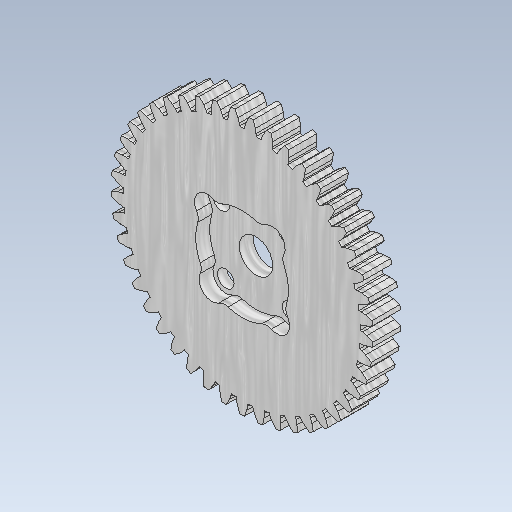
# Autodesk Inventor part: m1歯数45同軸ギア5td6
Saved by Autodesk Inventor 2020.2 (Build 242310000, 310)
## iProperties
Created: 2020-02-29
Part Number: m1歯数45同軸ギア5td6
Material: アルミニウム 7075
Document SubType Name: Modeling
Designer: aoyam
Density: 2.81 g/cm^3
Appearance: サテン - ブラシ仕上げ 重厚
Author: aoyam
Autodesk Inventor part; units mm, degrees
ref_plane "YZ Plane" through (0, 0, 0) normal (1, 0, 0) x (0, 1, 0)
ref_plane "XZ Plane" through (0, 0, 0) normal (0, 1, 0) x (-1, 0, 0)
ref_plane "XY Plane" through (0, 0, 0) normal (0, 0, 1) x (1, 0, 0)
sketch "スケッチ1" plane through (0, 0, 0) normal (0, 0, 1) x (1, 0, 0)
  arc A0 (1.8358, 22.8336) -> (1.7596, 22.4335) centre (5.1577, 21.9932) ccw
  arc A1 (2.0665, 23.5562) -> (1.8358, 22.8336) centre (7.6641, 21.3711) ccw
  arc A2 (2.5802, 24.6469) -> (2.0665, 23.5562) centre (10.2505, 20.3678) ccw
  arc A3 (0.898, 22.4335) -> (0.8218, 22.8336) centre (-2.5001, 21.9932) ccw
  arc A4 (0.8218, 22.8336) -> (0.5911, 23.5562) centre (-5.0065, 21.3711) ccw
  arc A5 (0.5911, 23.5562) -> (0.0774, 24.6469) centre (-7.5929, 20.3678) ccw
  arc A6 (1.7596, 22.4335) -> (0.898, 22.4335) centre (1.3288, 1.2587) ccw
  arc A7 (0.0774, 24.6469) -> (-0.687, 24.5934) centre (1.3288, 1.2587) ccw
  arc A8 (-1.1916, 22.2873) -> (-2.0447, 22.1674) centre (1.3288, 1.2587) ccw
  arc A9 (-2.0447, 22.1674) -> (-2.176, 22.5531) centre (-5.3485, 21.2585) ccw
  arc A10 (-1.1718, 22.6942) -> (-1.1916, 22.2873) centre (2.2347, 22.3243) ccw
  arc A11 (-2.176, 22.5531) -> (-2.505, 23.2366) centre (-7.744, 20.2937) ccw
  arc A12 (-1.0439, 23.4419) -> (-1.1718, 22.6942) centre (4.8033, 22.0571) ccw
  arc A13 (-0.687, 24.5934) -> (-1.0439, 23.4419) centre (7.5042, 21.4234) ccw
  arc A14 (-2.505, 23.2366) -> (-3.1655, 24.2451) centre (-10.1655, 18.9401) ccw
  arc A15 (-3.1655, 24.2451) -> (-3.9149, 24.0858) centre (1.3288, 1.2587) ccw
  arc A16 (-4.0937, 21.7319) -> (-4.9218, 21.4944) centre (1.3288, 1.2587) ccw
  arc A17 (-4.9218, 21.4944) -> (-5.1055, 21.8581) centre (-8.0669, 20.1346) ccw
  arc A18 (-4.1307, 22.1376) -> (-4.0937, 21.7319) centre (-0.7059, 22.2453) ccw
  arc A19 (-5.1055, 21.8581) -> (-5.5264, 22.4891) centre (-10.3048, 18.8457) ccw
  arc A20 (-4.1081, 22.8958) -> (-4.1307, 22.1376) centre (1.8749, 22.3382) ccw
  arc A21 (-3.9149, 24.0858) -> (-4.1081, 22.8958) centre (4.6377, 22.0867) ccw
  arc A22 (-5.5264, 22.4891) -> (-6.3208, 23.3959) centre (-12.5145, 17.1684) ccw
  arc A23 (-6.3208, 23.3959) -> (-7.0408, 23.1339) centre (1.3288, 1.2587) ccw
  arc A24 (-6.8902, 20.778) -> (-7.6773, 20.4276) centre (1.3288, 1.2587) ccw
  arc A25 (-7.6773, 20.4276) -> (-7.9097, 20.7621) centre (-10.6025, 18.6432) ccw
  arc A26 (-6.9833, 21.1746) -> (-6.8902, 20.778) centre (-3.6069, 21.7579) ccw
  arc A27 (-7.9097, 20.7621) -> (-8.4144, 21.3284) centre (-12.6393, 17.0555) ccw
  arc A28 (-7.0665, 21.9286) -> (-6.9833, 21.1746) centre (-1.0641, 22.2091) ccw
  arc A29 (-7.0408, 23.1339) -> (-7.0665, 21.9286) centre (1.7068, 22.3445) ccw
  arc A30 (-8.4144, 21.3284) -> (-9.3273, 22.1159) centre (-14.5939, 15.0869) ccw
  arc A31 (-9.3273, 22.1159) -> (-10.0038, 21.7562) centre (1.3288, 1.2587) ccw
  arc A32 (-9.5268, 19.4442) -> (-10.2574, 18.9876) centre (1.3288, 1.2587) ccw
  arc A33 (-10.2574, 18.9876) -> (-10.5342, 19.2866) centre (-12.9059, 16.8135) ccw
  arc A34 (-9.6742, 19.824) -> (-9.5268, 19.4442) centre (-6.4118, 20.8715) ccw
  arc A35 (-10.5342, 19.2866) -> (-11.1127, 19.7771) centre (-14.7018, 14.9578) ccw
  arc A36 (-9.8615, 20.559) -> (-9.6742, 19.824) centre (-3.9565, 21.6722) ccw
  arc A37 (-10.0038, 21.7562) -> (-9.8615, 20.559) centre (-1.2315, 22.1919) ccw
  arc A38 (-11.1127, 19.7771) -> (-12.1263, 20.4298) centre (-16.3635, 12.7363) ccw
  arc A39 (-12.1263, 20.4298) -> (-12.7462, 19.9795) centre (1.3288, 1.2587) ccw
  arc A40 (-11.9521, 17.7564) -> (-12.6121, 17.2026) centre (1.3288, 1.2587) ccw
  arc A41 (-12.6121, 17.2026) -> (-12.9277, 17.4601) centre (-14.9322, 14.6811) ccw
  arc A42 (-12.1509, 18.112) -> (-11.9521, 17.7564) centre (-9.066, 19.6034) ccw
  arc A43 (-12.9277, 17.4601) -> (-13.5689, 17.8654) centre (-16.4524, 12.5934) ccw
  arc A44 (-12.4387, 18.8138) -> (-12.1509, 18.112) centre (-6.7461, 20.7379) ccw
  arc A45 (-12.7462, 19.9795) -> (-12.4387, 18.8138) centre (-4.1199, 21.6318) ccw
  arc A46 (-13.5689, 17.8654) -> (-14.6635, 18.3707) centre (-17.7887, 10.1623) ccw
  arc A47 (-14.6635, 18.3707) -> (-15.2147, 17.8384) centre (1.3288, 1.2587) ccw
  arc A48 (-14.1189, 15.7475) -> (-14.6954, 15.1072) centre (1.3288, 1.2587) ccw
  arc A49 (-14.6954, 15.1072) -> (-15.0438, 15.3183) centre (-16.642, 12.2874) ccw
  arc A50 (-14.3653, 16.0719) -> (-14.1189, 15.7475) centre (-11.5179, 17.9782) ccw
  arc A51 (-15.0438, 15.3183) -> (-15.7352, 15.6304) centre (-17.8568, 10.0085) ccw
  arc A52 (-14.7479, 16.7269) -> (-14.3653, 16.0719) centre (-9.3785, 19.4246) ccw
  arc A53 (-15.2147, 17.8384) -> (-14.7479, 16.7269) centre (-6.9023, 20.6752) ccw
  arc A54 (-15.7352, 15.6304) -> (-16.8894, 15.9784) centre (-18.8418, 7.415) ccw
  arc A55 (-16.8894, 15.9784) -> (-17.3611, 15.3747) centre (1.3288, 1.2587) ccw
  arc A56 (-15.985, 13.4566) -> (-16.4668, 12.7423) centre (1.3288, 1.2587) ccw
  arc A57 (-16.4668, 12.7423) -> (-16.8412, 12.9029) centre (-18.002, 9.679) ccw
  arc A58 (-16.2741, 13.7436) -> (-15.985, 13.4566) centre (-13.7198, 16.0275) ccw
  arc A59 (-16.8412, 12.9029) -> (-17.5693, 13.1157) centre (-18.8878, 7.2532) ccw
  arc A60 (-16.7442, 14.3389) -> (-16.2741, 13.7436) centre (-11.8025, 17.7576) ccw
  arc A61 (-17.3611, 15.3747) -> (-16.7442, 14.3389) centre (-9.5244, 19.3407) ccw
  arc A62 (-17.5693, 13.1157) -> (-18.7607, 13.2997) centre (-19.5023, 4.5479) ccw
  arc A63 (-18.7607, 13.2997) -> (-19.1438, 12.6362) centre (1.3288, 1.2587) ccw
  arc A64 (-17.5141, 10.9283) -> (-17.8918, 10.1539) centre (1.3288, 1.2587) ccw
  arc A65 (-17.8918, 10.1539) -> (-18.2849, 10.2608) centre (-18.9857, 6.9067) ccw
  arc A66 (-17.8404, 11.1722) -> (-17.5141, 10.9283) centre (-15.6288, 13.7894) ccw
  arc A67 (-18.2849, 10.2608) -> (-19.0355, 10.3702) centre (-19.5254, 4.3812) ccw
  arc A68 (-18.3887, 11.6963) -> (-17.8404, 11.1722) centre (-13.9709, 15.7695) ccw
  arc A69 (-19.1438, 12.6362) -> (-18.3887, 11.6963) centre (-11.9353, 17.6543) ccw
  arc A70 (-19.0355, 10.3702) -> (-20.241, 10.3866) centre (-19.7574, 1.6168) ccw
  arc A71 (-20.241, 10.3866) -> (-20.528, 9.6762) centre (1.3288, 1.2587) ccw
  arc A72 (-18.6765, 8.2117) -> (-18.9427, 7.3924) centre (1.3288, 1.2587) ccw
  arc A73 (-18.9427, 7.3924) -> (-19.3469, 7.4435) centre (-19.5741, 4.0245) ccw
  arc A74 (-19.0335, 8.4079) -> (-18.6765, 8.2117) centre (-17.2077, 11.3074) ccw
  arc A75 (-19.3469, 7.4435) -> (-20.1054, 7.4474) centre (-19.757, 1.4485) ccw
  arc A76 (-19.6495, 8.8506) -> (-19.0335, 8.4079) centre (-15.8415, 13.499) ccw
  arc A77 (-20.528, 9.6762) -> (-19.6495, 8.8506) centre (-14.0881, 15.6487) ccw
  arc A78 (-20.1054, 7.4474) -> (-21.3014, 7.2958) centre (-19.602, -1.3213) ccw
  arc A79 (-21.3014, 7.2958) -> (-21.4868, 6.5524) centre (1.3288, 1.2587) ccw
  arc A80 (-19.4495, 5.3599) -> (-19.5991, 4.5114) centre (1.3288, 1.2587) ccw
  arc A81 (-19.5991, 4.5114) -> (-20.0064, 4.5058) centre (-19.7556, 1.0885) ccw
  arc A82 (-19.8303, 5.5044) -> (-19.4495, 5.3599) centre (-18.4258, 8.6299) ccw
  arc A83 (-20.0064, 4.5058) -> (-20.7581, 4.4041) centre (-19.5782, -1.4879) ccw
  arc A84 (-20.5019, 5.8571) -> (-19.8303, 5.5044) centre (-17.378, 10.9902) ccw
  arc A85 (-21.4868, 6.5524) -> (-20.5019, 5.8571) centre (-15.9408, 13.3631) ccw
  arc A86 (-20.7581, 4.4041) -> (-21.9214, 4.0876) centre (-19.0392, -4.2092) ccw
  arc A87 (-21.9214, 4.0876) -> (-22.0015, 3.3256) centre (1.3288, 1.2587) ccw
  arc A88 (-19.8181, 2.4282) -> (-19.8481, 1.5672) centre (1.3288, 1.2587) ccw
  arc A89 (-19.8481, 1.5672) -> (-20.2507, 1.5049) centre (-19.5267, -1.8442) ccw
  arc A90 (-20.2153, 2.5183) -> (-19.8181, 2.4282) centre (-19.2595, 5.8088) ccw
  arc A91 (-20.2507, 1.5049) -> (-20.9809, 1.2996) centre (-18.9925, -4.3709) ccw
  arc A92 (-20.9294, 2.7741) -> (-20.2153, 2.5183) centre (-18.5503, 8.292) ccw
  arc A93 (-22.0015, 3.3256) -> (-20.9294, 2.7741) centre (-17.4573, 10.8418) ccw
  arc A94 (-20.9809, 1.2996) -> (-22.0888, 0.8242) centre (-18.08, -6.9907) ccw
  arc A95 (-22.0888, 0.8242) -> (-22.0621, 0.0585) centre (1.3288, 1.2587) ccw
  arc A96 (-19.775, -0.5263) -> (-19.685, -1.3831) centre (1.3288, 1.2587) ccw
  arc A97 (-19.685, -1.3831) -> (-20.075, -1.5008) centre (-18.8919, -4.7166) ccw
  arc A98 (-20.181, -0.4923) -> (-19.775, -0.5263) centre (-19.6924, 2.8992) ccw
  arc A99 (-20.075, -1.5008) -> (-20.7695, -1.8057) centre (-18.0112, -7.1443) ccw
  arc A100 (-20.9237, -0.3384) -> (-20.181, -0.4923) centre (-19.3357, 5.4569) ccw
  arc A101 (-22.0621, 0.0585) -> (-20.9237, -0.3384) centre (-18.6082, 8.134) ccw
  arc A102 (-20.7695, -1.8057) -> (-21.8005, -2.4306) centre (-16.743, -9.6116) ccw
  arc A103 (-21.8005, -2.4306) -> (-21.6674, -3.1852) centre (1.3288, 1.2587) ccw
  arc A104 (-19.3212, -3.446) -> (-19.1128, -4.2819) centre (1.3288, 1.2587) ccw
  arc A105 (-19.1128, -4.2819) -> (-19.4826, -4.4528) centre (-17.8635, -7.4726) ccw
  arc A106 (-19.728, -3.4688) -> (-19.3212, -3.446) centre (-19.7161, -0.0423) ccw
  arc A107 (-19.4826, -4.4528) -> (-20.128, -4.8514) centre (-16.6536, -9.7541) ccw
  arc A108 (-20.4849, -3.4198) -> (-19.728, -3.4688) centre (-19.7189, 2.5401) ccw
  arc A109 (-21.6674, -3.1852) -> (-20.4849, -3.4198) centre (-19.371, 5.2924) ccw
  arc A110 (-20.128, -4.8514) -> (-21.0619, -5.6137) centre (-15.0543, -12.0209) ccw
  arc A111 (-21.0619, -5.6137) -> (-20.8252, -6.3424) centre (1.3288, 1.2587) ccw
  arc A112 (-18.4655, -6.2741) -> (-18.1428, -7.0729) centre (1.3288, 1.2587) ccw
  arc A113 (-18.1428, -7.0729) -> (-18.4852, -7.2936) centre (-16.4616, -10.0587) ccw
  arc A114 (-18.8651, -6.3533) -> (-18.4655, -6.2741) centre (-19.3302, -2.9586) ccw
  arc A115 (-18.4852, -7.2936) -> (-19.0688, -7.7782) centre (-14.9459, -12.1496) ccw
  arc A116 (-19.6215, -6.4101) -> (-18.8651, -6.3533) centre (-19.6924, -0.4016) ccw
  arc A117 (-20.8252, -6.3424) -> (-19.6215, -6.4101) centre (-19.731, 2.3723) ccw
  arc A118 (-19.0688, -7.7782) -> (-19.8876, -8.663) centre (-13.0467, -14.1718) ccw
  arc A119 (-19.8876, -8.663) -> (-19.5517, -9.3517) centre (1.3288, 1.2587) ccw
  arc A120 (-17.2245, -8.9557) -> (-16.7937, -9.7018) centre (1.3288, 1.2587) ccw
  arc A121 (-16.7937, -9.7018) -> (-17.1022, -9.9679) centre (-14.7134, -12.4245) ccw
  arc A122 (-17.6092, -9.0897) -> (-17.2245, -8.9557) centre (-18.5422, -5.7927) ccw
  arc A123 (-17.1022, -9.9679) -> (-17.6126, -10.529) centre (-12.9214, -14.2841) ccw
  arc A124 (-18.3503, -9.2512) -> (-17.6092, -9.0897) centre (-19.2567, -3.311) ccw
  arc A125 (-19.5517, -9.3517) -> (-18.3503, -9.2512) centre (-19.681, -0.5695) ccw
  arc A126 (-17.6126, -10.529) -> (-18.3003, -11.5192) centre (-10.7593, -16.0223) ccw
  arc A127 (-18.3003, -11.5192) -> (-17.8718, -12.1544) centre (1.3288, 1.2587) ccw
  arc A128 (-15.6224, -11.4384) -> (-15.092, -12.1173) centre (1.3288, 1.2587) ccw
  arc A129 (-15.092, -12.1173) -> (-15.3603, -12.4238) centre (-12.6529, -14.524) ccw
  arc A130 (-15.9847, -11.6247) -> (-15.6224, -11.4384) centre (-17.3675, -8.4896) ccw
  arc A131 (-15.3603, -12.4238) -> (-15.7877, -13.0504) centre (-10.6196, -16.1161) ccw
  arc A132 (-16.6961, -11.8878) -> (-15.9847, -11.6247) centre (-18.4204, -6.1315) ccw
  arc A133 (-17.8718, -12.1544) -> (-16.6961, -11.8878) centre (-19.2221, -3.4757) ccw
  arc A134 (-15.7877, -13.0504) -> (-16.3309, -14.1267) centre (-8.2366, -17.5364) ccw
  arc A135 (-16.3309, -14.1267) -> (-15.8182, -14.6961) centre (1.3288, 1.2587) ccw
  arc A136 (-13.6903, -13.674) -> (-13.0706, -14.2724) centre (1.3288, 1.2587) ccw
  arc A137 (-13.0706, -14.2724) -> (-13.2937, -14.6133) centre (-10.3204, -16.3162) ccw
  arc A138 (-14.0232, -13.9088) -> (-13.6903, -13.674) centre (-15.8289, -10.9967) ccw
  arc A139 (-13.2937, -14.6133) -> (-13.6297, -15.2933) centre (-8.0852, -17.6099) ccw
  arc A140 (-14.6911, -14.2684) -> (-14.0232, -13.9088) centre (-17.1997, -8.8081) ccw
  arc A141 (-15.8182, -14.6961) -> (-14.6911, -14.2684) centre (-18.3632, -6.2897) ccw
  arc A142 (-13.6297, -15.2933) -> (-14.0178, -16.4347) centre (-5.5278, -18.6848) ccw
  arc A143 (-14.0178, -16.4347) -> (-13.4309, -16.9272) centre (1.3288, 1.2587) ccw
  arc A144 (-11.4659, -15.6189) -> (-10.7689, -16.1253) centre (1.3288, 1.2587) ccw
  arc A145 (-10.7689, -16.1253) -> (-10.9425, -16.4939) centre (-7.761, -17.7664) ccw
  arc A146 (-11.7628, -15.8978) -> (-11.4659, -15.6189) centre (-13.9563, -13.2654) ccw
  arc A147 (-10.9425, -16.4939) -> (-11.1806, -17.2141) centre (-5.3676, -18.7364) ccw
  arc A148 (-12.3742, -16.3468) -> (-11.7628, -15.8978) centre (-15.6184, -11.2888) ccw
  arc A149 (-13.4309, -16.9272) -> (-12.3742, -16.3468) centre (-17.121, -8.9569) ccw
  arc A150 (-11.1806, -17.2141) -> (-11.406, -18.3984) centre (-2.6855, -19.4449) ccw
  arc A151 (-11.406, -18.3984) -> (-10.7563, -18.8044) centre (1.3288, 1.2587) ccw
  arc A152 (-8.9925, -17.2353) -> (-8.2318, -17.6398) centre (1.3288, 1.2587) ccw
  arc A153 (-8.2318, -17.6398) -> (-8.3524, -18.0289) centre (-5.0248, -18.8464) ccw
  arc A154 (-9.2477, -17.5529) -> (-8.9925, -17.2353) centre (-11.7861, -15.2513) ccw
  arc A155 (-8.3524, -18.0289) -> (-8.4879, -18.7753) centre (-2.5197, -19.4738) ccw
  arc A156 (-9.7906, -18.0826) -> (-9.2477, -17.5529) centre (-13.7072, -13.5253) ccw
  arc A157 (-10.7563, -18.8044) -> (-9.7906, -18.0826) centre (-15.5198, -11.4252) ccw
  arc A158 (-8.4879, -18.7753) -> (-8.5464, -19.9794) centre (0.235, -19.8021) ccw
  arc A159 (-8.5464, -19.9794) -> (-7.8464, -20.291) centre (1.3288, 1.2587) ccw
  arc A160 (-6.3182, -18.4918) -> (-5.5086, -18.7865) centre (1.3288, 1.2587) ccw
  arc A161 (-5.5086, -18.7865) -> (-5.5738, -19.1886) centre (-2.1649, -19.5349) ccw
  arc A162 (-6.5267, -18.8417) -> (-6.3182, -18.4918) centre (-9.3608, -16.9159) ccw
  arc A163 (-5.5738, -19.1886) -> (-5.6042, -19.9465) centre (0.4032, -19.8076) ccw
  arc A164 (-6.9907, -19.4419) -> (-6.5267, -18.8417) centre (-11.5033, -15.474) ccw
  arc A165 (-7.8464, -20.291) -> (-6.9907, -19.4419) centre (-13.5905, -13.6466) ccw
  arc A166 (-5.6042, -19.9465) -> (-5.4945, -21.1471) centre (3.1767, -19.7494) ccw
  arc A167 (-5.4945, -21.1471) -> (-4.758, -21.3583) centre (1.3288, 1.2587) ccw
  arc A168 (-3.495, -19.3638) -> (-2.6523, -19.543) centre (1.3288, 1.2587) ccw
  arc A169 (-2.6523, -19.543) -> (-2.6609, -19.9502) centre (0.763, -19.8188) ccw
  arc A170 (-3.6528, -19.7394) -> (-3.495, -19.3638) centre (-6.7273, -18.2267) ccw
  arc A171 (-2.6609, -19.9502) -> (-2.5855, -20.705) centre (3.344, -19.7314) ccw
  arc A172 (-4.0287, -20.3983) -> (-3.6528, -19.7394) centre (-9.0497, -17.0971) ccw
  arc A173 (-4.758, -21.3583) -> (-4.0287, -20.3983) centre (-11.3709, -15.5779) ccw
  arc A174 (-2.5855, -20.705) -> (-2.3098, -21.8786) centre (6.0825, -19.2878) ccw
  arc A175 (-2.3098, -21.8786) -> (-1.5511, -21.9853) centre (1.3288, 1.2587) ccw
  arc A176 (-0.578, -19.8345) -> (0.2814, -19.8946) centre (1.3288, 1.2587) ccw
  arc A177 (0.2814, -19.8946) -> (0.3296, -20.2991) centre (3.702, -19.6924) ccw
  arc A178 (-0.682, -20.2284) -> (-0.578, -19.8345) centre (-3.9371, -19.1582) ccw
  arc A179 (0.3296, -20.2991) -> (0.5093, -21.036) centre (6.2457, -19.2467) ccw
  arc A180 (-0.9625, -20.9331) -> (-0.682, -20.2284) centre (-6.394, -18.3628) ccw
  arc A181 (-1.5511, -21.9853) -> (-0.9625, -20.9331) centre (-8.9041, -17.1815) ccw
  arc A182 (0.5093, -21.036) -> (0.9457, -22.1599) centre (8.8958, -18.4262) ccw
  arc A183 (0.9457, -22.1599) -> (1.7119, -22.1599) centre (1.3288, 1.2587) ccw
  arc A184 (2.3762, -19.8946) -> (3.2356, -19.8345) centre (1.3288, 1.2587) ccw
  arc A185 (3.2356, -19.8345) -> (3.3396, -20.2284) centre (6.5947, -19.1582) ccw
  arc A186 (2.328, -20.2991) -> (2.3762, -19.8946) centre (-1.0444, -19.6924) ccw
  arc A187 (3.3396, -20.2284) -> (3.6201, -20.9331) centre (9.0516, -18.3628) ccw
  arc A188 (2.1483, -21.036) -> (2.328, -20.2991) centre (-3.5881, -19.2467) ccw
  arc A189 (1.7119, -22.1599) -> (2.1483, -21.036) centre (-6.2382, -18.4262) ccw
  arc A190 (3.6201, -20.9331) -> (4.2087, -21.9853) centre (11.5617, -17.1815) ccw
  arc A191 (4.2087, -21.9853) -> (4.9674, -21.8786) centre (1.3288, 1.2587) ccw
  arc A192 (5.3099, -19.543) -> (6.1526, -19.3638) centre (1.3288, 1.2587) ccw
  arc A193 (6.1526, -19.3638) -> (6.3104, -19.7394) centre (9.3849, -18.2267) ccw
  arc A194 (5.3185, -19.9502) -> (5.3099, -19.543) centre (1.8946, -19.8188) ccw
  arc A195 (6.3104, -19.7394) -> (6.6863, -20.3983) centre (11.7073, -17.0971) ccw
  arc A196 (5.2431, -20.705) -> (5.3185, -19.9502) centre (-0.6865, -19.7314) ccw
  arc A197 (4.9674, -21.8786) -> (5.2431, -20.705) centre (-3.4249, -19.2878) ccw
  arc A198 (6.6863, -20.3983) -> (7.4156, -21.3583) centre (14.0285, -15.5779) ccw
  arc A199 (7.4156, -21.3583) -> (8.1521, -21.1471) centre (1.3288, 1.2587) ccw
  arc A200 (8.1662, -18.7865) -> (8.9758, -18.4918) centre (1.3288, 1.2587) ccw
  arc A201 (8.9758, -18.4918) -> (9.1843, -18.8417) centre (12.0184, -16.9159) ccw
  arc A202 (8.2314, -19.1886) -> (8.1662, -18.7865) centre (4.8225, -19.5349) ccw
  arc A203 (9.1843, -18.8417) -> (9.6482, -19.4419) centre (14.1609, -15.474) ccw
  arc A204 (8.2618, -19.9465) -> (8.2314, -19.1886) centre (2.2544, -19.8076) ccw
  arc A205 (8.1521, -21.1471) -> (8.2618, -19.9465) centre (-0.5191, -19.7494) ccw
  arc A206 (9.6482, -19.4419) -> (10.504, -20.291) centre (16.2481, -13.6466) ccw
  arc A207 (10.504, -20.291) -> (11.2039, -19.9794) centre (1.3288, 1.2587) ccw
  arc A208 (10.8894, -17.6398) -> (11.6501, -17.2353) centre (1.3288, 1.2587) ccw
  arc A209 (11.6501, -17.2353) -> (11.9053, -17.5529) centre (14.4437, -15.2513) ccw
  arc A210 (11.0099, -18.0289) -> (10.8894, -17.6398) centre (7.6824, -18.8464) ccw
  arc A211 (11.9053, -17.5529) -> (12.4482, -18.0826) centre (16.3648, -13.5253) ccw
  arc A212 (11.1455, -18.7753) -> (11.0099, -18.0289) centre (5.1773, -19.4738) ccw
  arc A213 (11.2039, -19.9794) -> (11.1455, -18.7753) centre (2.4226, -19.8021) ccw
  arc A214 (12.4482, -18.0826) -> (13.4138, -18.8044) centre (18.1773, -11.4252) ccw
  arc A215 (13.4138, -18.8044) -> (14.0636, -18.3984) centre (1.3288, 1.2587) ccw
  arc A216 (13.4265, -16.1253) -> (14.1235, -15.6189) centre (1.3288, 1.2587) ccw
  arc A217 (14.1235, -15.6189) -> (14.4204, -15.8978) centre (16.6138, -13.2654) ccw
  arc A218 (13.6, -16.4939) -> (13.4265, -16.1253) centre (10.4186, -17.7664) ccw
  arc A219 (14.4204, -15.8978) -> (15.0318, -16.3468) centre (18.276, -11.2888) ccw
  arc A220 (13.8381, -17.2141) -> (13.6, -16.4939) centre (8.0252, -18.7364) ccw
  arc A221 (14.0636, -18.3984) -> (13.8381, -17.2141) centre (5.343, -19.4449) ccw
  arc A222 (15.0318, -16.3468) -> (16.0885, -16.9272) centre (19.7786, -8.9569) ccw
  arc A223 (16.0885, -16.9272) -> (16.6754, -16.4347) centre (1.3288, 1.2587) ccw
  arc A224 (15.7282, -14.2724) -> (16.3479, -13.674) centre (1.3288, 1.2587) ccw
  arc A225 (16.3479, -13.674) -> (16.6807, -13.9088) centre (18.4864, -10.9967) ccw
  arc A226 (15.9513, -14.6133) -> (15.7282, -14.2724) centre (12.9779, -16.3162) ccw
  arc A227 (16.6807, -13.9088) -> (17.3487, -14.2684) centre (19.8573, -8.8081) ccw
  arc A228 (16.2873, -15.2933) -> (15.9513, -14.6133) centre (10.7428, -17.6099) ccw
  arc A229 (16.6754, -16.4347) -> (16.2873, -15.2933) centre (8.1854, -18.6848) ccw
  arc A230 (17.3487, -14.2684) -> (18.4758, -14.6961) centre (21.0208, -6.2897) ccw
  arc A231 (18.4758, -14.6961) -> (18.9885, -14.1267) centre (1.3288, 1.2587) ccw
  arc A232 (17.7495, -12.1173) -> (18.28, -11.4384) centre (1.3288, 1.2587) ccw
  arc A233 (18.28, -11.4384) -> (18.6423, -11.6247) centre (20.0251, -8.4896) ccw
  arc A234 (18.0179, -12.4238) -> (17.7495, -12.1173) centre (15.3105, -14.524) ccw
  arc A235 (18.6423, -11.6247) -> (19.3537, -11.8878) centre (21.078, -6.1315) ccw
  arc A236 (18.4453, -13.0504) -> (18.0179, -12.4238) centre (13.2772, -16.1161) ccw
  arc A237 (18.9885, -14.1267) -> (18.4453, -13.0504) centre (10.8942, -17.5364) ccw
  arc A238 (19.3537, -11.8878) -> (20.5294, -12.1544) centre (21.8797, -3.4757) ccw
  arc A239 (20.5294, -12.1544) -> (20.9579, -11.5192) centre (1.3288, 1.2587) ccw
  arc A240 (19.4513, -9.7018) -> (19.8821, -8.9557) centre (1.3288, 1.2587) ccw
  arc A241 (19.8821, -8.9557) -> (20.2668, -9.0897) centre (21.1998, -5.7927) ccw
  arc A242 (19.7597, -9.9679) -> (19.4513, -9.7018) centre (17.371, -12.4245) ccw
  arc A243 (20.2668, -9.0897) -> (21.0079, -9.2512) centre (21.9143, -3.311) ccw
  arc A244 (20.2702, -10.529) -> (19.7597, -9.9679) centre (15.579, -14.2841) ccw
  arc A245 (20.9579, -11.5192) -> (20.2702, -10.529) centre (13.4169, -16.0223) ccw
  arc A246 (21.0079, -9.2512) -> (22.2093, -9.3517) centre (22.3386, -0.5695) ccw
  arc A247 (22.2093, -9.3517) -> (22.5452, -8.663) centre (1.3288, 1.2587) ccw
  arc A248 (20.8003, -7.0729) -> (21.1231, -6.2741) centre (1.3288, 1.2587) ccw
  arc A249 (21.1231, -6.2741) -> (21.5227, -6.3533) centre (21.9878, -2.9586) ccw
  arc A250 (21.1428, -7.2936) -> (20.8003, -7.0729) centre (19.1192, -10.0587) ccw
  arc A251 (21.5227, -6.3533) -> (22.2791, -6.4101) centre (22.35, -0.4016) ccw
  arc A252 (21.7264, -7.7782) -> (21.1428, -7.2936) centre (17.6035, -12.1496) ccw
  arc A253 (22.5452, -8.663) -> (21.7264, -7.7782) centre (15.7043, -14.1718) ccw
  arc A254 (22.2791, -6.4101) -> (23.4828, -6.3424) centre (22.3886, 2.3723) ccw
  arc A255 (23.4828, -6.3424) -> (23.7195, -5.6137) centre (1.3288, 1.2587) ccw
  arc A256 (21.7704, -4.2819) -> (21.9788, -3.446) centre (1.3288, 1.2587) ccw
  arc A257 (21.9788, -3.446) -> (22.3855, -3.4688) centre (22.3737, -0.0423) ccw
  arc A258 (22.1402, -4.4528) -> (21.7704, -4.2819) centre (20.5211, -7.4726) ccw
  arc A259 (22.3855, -3.4688) -> (23.1425, -3.4198) centre (22.3765, 2.5401) ccw
  arc A260 (22.7856, -4.8514) -> (22.1402, -4.4528) centre (19.3112, -9.7541) ccw
  arc A261 (23.7195, -5.6137) -> (22.7856, -4.8514) centre (17.7119, -12.0209) ccw
  arc A262 (23.1425, -3.4198) -> (24.325, -3.1852) centre (22.0286, 5.2924) ccw
  arc A263 (24.325, -3.1852) -> (24.4581, -2.4306) centre (1.3288, 1.2587) ccw
  arc A264 (22.3426, -1.3831) -> (22.4326, -0.5263) centre (1.3288, 1.2587) ccw
  arc A265 (22.4326, -0.5263) -> (22.8386, -0.4923) centre (22.3499, 2.8992) ccw
  arc A266 (22.7326, -1.5008) -> (22.3426, -1.3831) centre (21.5495, -4.7166) ccw
  arc A267 (22.8386, -0.4923) -> (23.5813, -0.3384) centre (21.9933, 5.4569) ccw
  arc A268 (23.4271, -1.8057) -> (22.7326, -1.5008) centre (20.6688, -7.1443) ccw
  arc A269 (24.4581, -2.4306) -> (23.4271, -1.8057) centre (19.4006, -9.6116) ccw
  arc A270 (23.5813, -0.3384) -> (24.7197, 0.0585) centre (21.2658, 8.134) ccw
  arc A271 (24.7197, 0.0585) -> (24.7464, 0.8242) centre (1.3288, 1.2587) ccw
  arc A272 (22.5057, 1.5672) -> (22.4756, 2.4282) centre (1.3288, 1.2587) ccw
  arc A273 (22.4756, 2.4282) -> (22.8729, 2.5183) centre (21.917, 5.8088) ccw
  arc A274 (22.9083, 1.5049) -> (22.5057, 1.5672) centre (22.1843, -1.8442) ccw
  arc A275 (22.8729, 2.5183) -> (23.587, 2.7741) centre (21.2079, 8.292) ccw
  arc A276 (23.6385, 1.2996) -> (22.9083, 1.5049) centre (21.6501, -4.3709) ccw
  arc A277 (24.7464, 0.8242) -> (23.6385, 1.2996) centre (20.7376, -6.9907) ccw
  arc A278 (23.587, 2.7741) -> (24.6591, 3.3256) centre (20.1149, 10.8418) ccw
  arc A279 (24.6591, 3.3256) -> (24.579, 4.0876) centre (1.3288, 1.2587) ccw
  arc A280 (22.2567, 4.5114) -> (22.1071, 5.3599) centre (1.3288, 1.2587) ccw
  arc A281 (22.1071, 5.3599) -> (22.4879, 5.5044) centre (21.0834, 8.6299) ccw
  arc A282 (22.664, 4.5058) -> (22.2567, 4.5114) centre (22.4132, 1.0885) ccw
  arc A283 (22.4879, 5.5044) -> (23.1595, 5.8571) centre (20.0356, 10.9902) ccw
  arc A284 (23.4157, 4.4041) -> (22.664, 4.5058) centre (22.2358, -1.4879) ccw
  arc A285 (24.579, 4.0876) -> (23.4157, 4.4041) centre (21.6968, -4.2092) ccw
  arc A286 (23.1595, 5.8571) -> (24.1444, 6.5524) centre (18.5983, 13.3631) ccw
  arc A287 (24.1444, 6.5524) -> (23.959, 7.2958) centre (1.3288, 1.2587) ccw
  arc A288 (21.6003, 7.3924) -> (21.3341, 8.2117) centre (1.3288, 1.2587) ccw
  arc A289 (21.3341, 8.2117) -> (21.6911, 8.4079) centre (19.8653, 11.3074) ccw
  arc A290 (22.0045, 7.4435) -> (21.6003, 7.3924) centre (22.2317, 4.0245) ccw
  arc A291 (21.6911, 8.4079) -> (22.3071, 8.8506) centre (18.4991, 13.499) ccw
  arc A292 (22.763, 7.4474) -> (22.0045, 7.4435) centre (22.4146, 1.4485) ccw
  arc A293 (23.959, 7.2958) -> (22.763, 7.4474) centre (22.2596, -1.3213) ccw
  arc A294 (22.3071, 8.8506) -> (23.1856, 9.6762) centre (16.7457, 15.6487) ccw
  arc A295 (23.1856, 9.6762) -> (22.8986, 10.3866) centre (1.3288, 1.2587) ccw
  arc A296 (20.5494, 10.1539) -> (20.1717, 10.9283) centre (1.3288, 1.2587) ccw
  arc A297 (20.1717, 10.9283) -> (20.498, 11.1722) centre (18.2864, 13.7894) ccw
  arc A298 (20.9425, 10.2608) -> (20.5494, 10.1539) centre (21.6433, 6.9067) ccw
  arc A299 (20.498, 11.1722) -> (21.0463, 11.6963) centre (16.6285, 15.7695) ccw
  arc A300 (21.6931, 10.3702) -> (20.9425, 10.2608) centre (22.1829, 4.3812) ccw
  arc A301 (22.8986, 10.3866) -> (21.6931, 10.3702) centre (22.4149, 1.6168) ccw
  arc A302 (21.0463, 11.6963) -> (21.8014, 12.6362) centre (14.5929, 17.6543) ccw
  arc A303 (21.8014, 12.6362) -> (21.4183, 13.2997) centre (1.3288, 1.2587) ccw
  arc A304 (19.1244, 12.7423) -> (18.6426, 13.4566) centre (1.3288, 1.2587) ccw
  arc A305 (18.6426, 13.4566) -> (18.9317, 13.7436) centre (16.3774, 16.0275) ccw
  arc A306 (19.4988, 12.9029) -> (19.1244, 12.7423) centre (20.6596, 9.679) ccw
  arc A307 (18.9317, 13.7436) -> (19.4018, 14.3389) centre (14.4601, 17.7576) ccw
  arc A308 (20.2268, 13.1157) -> (19.4988, 12.9029) centre (21.5454, 7.2532) ccw
  arc A309 (21.4183, 13.2997) -> (20.2268, 13.1157) centre (22.1599, 4.5479) ccw
  arc A310 (19.4018, 14.3389) -> (20.0187, 15.3747) centre (12.182, 19.3407) ccw
  arc A311 (20.0187, 15.3747) -> (19.547, 15.9784) centre (1.3288, 1.2587) ccw
  arc A312 (17.353, 15.1072) -> (16.7765, 15.7475) centre (1.3288, 1.2587) ccw
  arc A313 (16.7765, 15.7475) -> (17.0228, 16.0719) centre (14.1755, 17.9782) ccw
  arc A314 (17.7014, 15.3183) -> (17.353, 15.1072) centre (19.2995, 12.2874) ccw
  arc A315 (17.0228, 16.0719) -> (17.4055, 16.7269) centre (12.0361, 19.4246) ccw
  arc A316 (18.3927, 15.6304) -> (17.7014, 15.3183) centre (20.5144, 10.0085) ccw
  arc A317 (19.547, 15.9784) -> (18.3927, 15.6304) centre (21.4994, 7.415) ccw
  arc A318 (17.4055, 16.7269) -> (17.8723, 17.8384) centre (9.5599, 20.6752) ccw
  arc A319 (17.8723, 17.8384) -> (17.3211, 18.3707) centre (1.3288, 1.2587) ccw
  arc A320 (15.2697, 17.2026) -> (14.6097, 17.7564) centre (1.3288, 1.2587) ccw
  arc A321 (14.6097, 17.7564) -> (14.8085, 18.112) centre (11.7236, 19.6034) ccw
  arc A322 (15.5853, 17.4601) -> (15.2697, 17.2026) centre (17.5898, 14.6811) ccw
  arc A323 (14.8085, 18.112) -> (15.0963, 18.8138) centre (9.4037, 20.7379) ccw
  arc A324 (16.2265, 17.8654) -> (15.5853, 17.4601) centre (19.1099, 12.5934) ccw
  arc A325 (17.3211, 18.3707) -> (16.2265, 17.8654) centre (20.4463, 10.1623) ccw
  arc A326 (15.0963, 18.8138) -> (15.4038, 19.9795) centre (6.7775, 21.6318) ccw
  arc A327 (15.4038, 19.9795) -> (14.7839, 20.4298) centre (1.3288, 1.2587) ccw
  arc A328 (12.915, 18.9876) -> (12.1844, 19.4442) centre (1.3288, 1.2587) ccw
  arc A329 (12.1844, 19.4442) -> (12.3318, 19.824) centre (9.0694, 20.8715) ccw
  arc A330 (13.1918, 19.2866) -> (12.915, 18.9876) centre (15.5635, 16.8135) ccw
  arc A331 (12.3318, 19.824) -> (12.5191, 20.559) centre (6.6141, 21.6722) ccw
  arc A332 (13.7703, 19.7771) -> (13.1918, 19.2866) centre (17.3594, 14.9578) ccw
  arc A333 (14.7839, 20.4298) -> (13.7703, 19.7771) centre (19.0211, 12.7363) ccw
  arc A334 (12.5191, 20.559) -> (12.6614, 21.7562) centre (3.8891, 22.1919) ccw
  arc A335 (12.6614, 21.7562) -> (11.9849, 22.1159) centre (1.3288, 1.2587) ccw
  arc A336 (10.3349, 20.4276) -> (9.5478, 20.778) centre (1.3288, 1.2587) ccw
  arc A337 (9.5478, 20.778) -> (9.6409, 21.1746) centre (6.2644, 21.7579) ccw
  arc A338 (10.5673, 20.7621) -> (10.3349, 20.4276) centre (13.2601, 18.6432) ccw
  arc A339 (9.6409, 21.1746) -> (9.7241, 21.9286) centre (3.7217, 22.2091) ccw
  arc A340 (11.072, 21.3284) -> (10.5673, 20.7621) centre (15.2968, 17.0555) ccw
  arc A341 (11.9849, 22.1159) -> (11.072, 21.3284) centre (17.2515, 15.0869) ccw
  arc A342 (9.7241, 21.9286) -> (9.6984, 23.1339) centre (0.9508, 22.3445) ccw
  arc A343 (9.6984, 23.1339) -> (8.9784, 23.3959) centre (1.3288, 1.2587) ccw
  arc A344 (7.5794, 21.4944) -> (6.7513, 21.7319) centre (1.3288, 1.2587) ccw
  arc A345 (6.7513, 21.7319) -> (6.7883, 22.1376) centre (3.3635, 22.2453) ccw
  arc A346 (7.7631, 21.8581) -> (7.5794, 21.4944) centre (10.7245, 20.1346) ccw
  arc A347 (6.7883, 22.1376) -> (6.7657, 22.8958) centre (0.7826, 22.3382) ccw
  arc A348 (8.184, 22.4891) -> (7.7631, 21.8581) centre (12.9624, 18.8457) ccw
  arc A349 (8.9784, 23.3959) -> (8.184, 22.4891) centre (15.172, 17.1684) ccw
  arc A350 (6.7657, 22.8958) -> (6.5725, 24.0858) centre (-1.9801, 22.0867) ccw
  arc A351 (6.5725, 24.0858) -> (5.8231, 24.2451) centre (1.3288, 1.2587) ccw
  arc A352 (4.7023, 22.1674) -> (3.8492, 22.2873) centre (1.3288, 1.2587) ccw
  arc A353 (3.8492, 22.2873) -> (3.8294, 22.6942) centre (0.4229, 22.3243) ccw
  arc A354 (4.8335, 22.5531) -> (4.7023, 22.1674) centre (8.0061, 21.2585) ccw
  arc A355 (3.8294, 22.6942) -> (3.7015, 23.4419) centre (-2.1457, 22.0571) ccw
  arc A356 (5.1626, 23.2366) -> (4.8335, 22.5531) centre (10.4016, 20.2937) ccw
  arc A357 (5.8231, 24.2451) -> (5.1626, 23.2366) centre (12.8231, 18.9401) ccw
  arc A358 (3.7015, 23.4419) -> (3.3446, 24.5934) centre (-4.8466, 21.4234) ccw
  arc A359 (3.3446, 24.5934) -> (2.5802, 24.6469) centre (1.3288, 1.2587) ccw
  circle A360 centre (1.3288, 1.2587) radius 2.99
  circle A361 centre (-4.8951, 6.674) radius 1.5
  arc A362 (-3.9314, 8.7072) -> (-6.7755, 5.4385) centre (-4.8951, 6.674) ccw
  arc A363 (-3.8116, 7.7114) -> (-5.7727, 5.4576) centre (1.3288, 1.2587) ccw construction
  arc A364 (-6.5395, 3.739) -> (-6.7755, 5.4385) centre (-8.447, 4.3403) ccw
  arc A365 (-3.9314, 8.7072) -> (-2.2156, 8.7085) centre (-3.0748, 10.5145) ccw
  arc A366 (-1.1516, -6.6096) -> (-2.8511, -6.8456) centre (-1.7529, -8.5171) ccw
  arc A367 (-6.1198, -4.0015) -> (-2.8511, -6.8456) centre (-4.0866, -4.9652) ccw
  circle A368 centre (-4.0866, -4.9652) radius 1.5
  arc A369 (-6.1198, -4.0015) -> (-6.121, -2.2857) centre (-7.9271, -3.1449) ccw
  arc A370 (9.1971, -1.2217) -> (9.4331, -2.9212) centre (11.1046, -1.823) ccw
  arc A371 (6.589, -6.1899) -> (9.4331, -2.9212) centre (7.5526, -4.1567) ccw
  circle A372 centre (7.5526, -4.1567) radius 1.5
  arc A373 (6.589, -6.1899) -> (4.8732, -6.1912) centre (5.7324, -7.9972) ccw
  arc A374 (3.8091, 9.127) -> (5.5087, 9.363) centre (4.4104, 11.0345) ccw
  arc A375 (8.7774, 6.5189) -> (5.5087, 9.363) centre (6.7442, 7.4825) ccw
  circle A376 centre (6.7442, 7.4825) radius 1.5
  arc A377 (8.7774, 6.5189) -> (8.7786, 4.803) centre (10.5846, 5.6623) ccw
  arc A378 (3.8091, 9.127) -> (-2.2156, 8.7085) centre (1.3288, 1.2587) ccw
  arc A379 (7.7816, 6.3991) -> (5.5277, 8.3602) centre (1.3288, 1.2587) ccw construction
  arc A380 (9.1971, -1.2217) -> (8.7786, 4.803) centre (1.3288, 1.2587) ccw
  arc A381 (6.4692, -5.1941) -> (8.4303, -2.9403) centre (1.3288, 1.2587) ccw construction
  arc A382 (-1.1516, -6.6096) -> (4.8732, -6.1912) centre (1.3288, 1.2587) ccw
  arc A383 (-6.5395, 3.739) -> (-6.121, -2.2857) centre (1.3288, 1.2587) ccw
  arc A384 (-5.124, -3.8818) -> (-2.8701, -5.8428) centre (1.3288, 1.2587) ccw construction
  arc A385 (-3.91, 8.7524) -> (-2.2371, 8.7536) centre (-3.0748, 10.5145) ccw
  arc A386 (-3.91, 8.7524) -> (-6.8173, 5.4111) centre (-4.8951, 6.674) ccw
  arc A387 (-6.5872, 3.7541) -> (-6.8173, 5.4111) centre (-8.447, 4.3403) ccw
  arc A388 (-6.5872, 3.7541) -> (-6.1662, -2.3072) centre (1.3288, 1.2587) ccw
  arc A389 (-6.1649, -3.9801) -> (-6.1662, -2.3072) centre (-7.9271, -3.1449) ccw
  arc A390 (-6.1649, -3.9801) -> (-2.8236, -6.8874) centre (-4.0866, -4.9652) ccw
  arc A391 (-1.1666, -6.6573) -> (-2.8236, -6.8874) centre (-1.7529, -8.5171) ccw
  arc A392 (-1.1666, -6.6573) -> (4.8946, -6.2363) centre (1.3288, 1.2587) ccw
  arc A393 (6.5676, -6.2351) -> (4.8946, -6.2363) centre (5.7324, -7.9972) ccw
  arc A394 (6.5676, -6.2351) -> (9.4749, -2.8937) centre (7.5526, -4.1567) ccw
  arc A395 (9.2448, -1.2367) -> (9.4749, -2.8937) centre (11.1046, -1.823) ccw
  arc A396 (9.2448, -1.2367) -> (8.8238, 4.8245) centre (1.3288, 1.2587) ccw
  arc A397 (8.8225, 6.4974) -> (8.8238, 4.8245) centre (10.5846, 5.6623) ccw
  arc A398 (8.8225, 6.4974) -> (5.4812, 9.4047) centre (6.7442, 7.4825) ccw
  arc A399 (3.8242, 9.1747) -> (5.4812, 9.4047) centre (4.4104, 11.0345) ccw
  arc A400 (3.8242, 9.1747) -> (-2.2371, 8.7536) centre (1.3288, 1.2587) ccw
  point P0 (0, 0)
  point P1 (-8.4144, 21.3284)
  point P2 (-9.3273, 22.1159)
  point P3 (-10.0038, 21.7562)
  point P4 (-9.8615, 20.559)
  point P5 (-9.6742, 19.824)
  point P6 (-9.5268, 19.4442)
  point P7 (-10.5342, 19.2866)
  point P8 (-11.1127, 19.7771)
  point P9 (-12.1263, 20.4298)
  point P10 (-12.7462, 19.9795)
  point P11 (-12.1509, 18.112)
  point P12 (-11.9521, 17.7564)
  point P13 (-12.6121, 17.2026)
  point P14 (-12.9277, 17.4601)
  point P15 (-13.5689, 17.8654)
  point P16 (-14.6635, 18.3707)
  point P17 (-15.2147, 17.8384)
  point P18 (-14.7479, 16.7269)
  point P19 (-14.3653, 16.0719)
  point P20 (-14.1189, 15.7475)
  point P21 (-14.6954, 15.1072)
  point P22 (-15.0438, 15.3183)
  point P23 (-15.7352, 15.6304)
  point P24 (-16.8894, 15.9784)
  point P25 (-17.3611, 15.3747)
  point P26 (-16.2741, 13.7436)
  point P27 (-15.985, 13.4566)
  point P28 (-16.4668, 12.7423)
  point P29 (-16.8412, 12.9029)
  point P30 (-17.5693, 13.1157)
  point P31 (-18.7607, 13.2997)
  point P32 (-19.1438, 12.6362)
  point P33 (-17.8404, 11.1722)
  point P34 (-17.5141, 10.9283)
  point P35 (-17.8918, 10.1539)
  point P36 (-18.2849, 10.2608)
  point P37 (-19.0355, 10.3702)
  point P38 (-20.241, 10.3866)
  point P39 (-20.528, 9.6762)
  point P40 (-19.6495, 8.8506)
  point P41 (-19.0335, 8.4079)
  point P42 (-18.6765, 8.2117)
  point P43 (-18.9427, 7.3924)
  point P44 (-19.3469, 7.4435)
  point P45 (-20.1054, 7.4474)
  point P46 (-21.3014, 7.2958)
  point P47 (-21.4868, 6.5524)
  point P48 (-20.5019, 5.8571)
  point P49 (-19.8303, 5.5044)
  point P50 (-19.4495, 5.3599)
  point P51 (-19.5991, 4.5114)
  point P52 (-20.0064, 4.5058)
  point P53 (-20.7581, 4.4041)
  point P54 (-21.9214, 4.0876)
  point P55 (-22.0015, 3.3256)
  point P56 (-20.9294, 2.7741)
  point P57 (-20.2153, 2.5183)
  point P58 (-19.8181, 2.4282)
  point P59 (-19.8481, 1.5672)
  point P60 (-20.2507, 1.5049)
  point P61 (-20.9809, 1.2996)
  point P62 (-22.0888, 0.8242)
  point P63 (-22.0621, 0.0585)
  point P64 (-20.9237, -0.3384)
  point P65 (-20.181, -0.4923)
  point P66 (-19.775, -0.5263)
  point P67 (-19.685, -1.3831)
  point P68 (-20.075, -1.5008)
  point P69 (-20.7695, -1.8057)
  point P70 (-21.8005, -2.4306)
  point P71 (-21.6674, -3.1852)
  point P72 (-20.4849, -3.4198)
  point P73 (-19.728, -3.4688)
  point P74 (-19.3212, -3.446)
  point P75 (-19.1128, -4.2819)
  point P76 (-19.4826, -4.4528)
  point P77 (-20.128, -4.8514)
  point P78 (-21.0619, -5.6137)
  point P79 (-20.8252, -6.3424)
  point P80 (-19.6215, -6.4101)
  point P81 (-18.8651, -6.3533)
  point P82 (-18.4655, -6.2741)
  point P83 (-18.1428, -7.0729)
  point P84 (-18.4852, -7.2936)
  point P85 (-19.0688, -7.7782)
  point P86 (-19.8876, -8.663)
  point P87 (-19.5517, -9.3517)
  point P88 (-18.3503, -9.2512)
  point P89 (-17.6092, -9.0897)
  point P90 (-17.2245, -8.9557)
  point P91 (-16.7937, -9.7018)
  point P92 (-17.1022, -9.9679)
  point P93 (-17.6126, -10.529)
  point P94 (-18.3003, -11.5192)
  point P95 (-17.8718, -12.1544)
  point P96 (-16.6961, -11.8878)
  point P97 (-15.9847, -11.6247)
  point P98 (-15.6224, -11.4384)
  point P99 (-15.092, -12.1173)
  point P100 (-15.3603, -12.4238)
  point P101 (-15.7877, -13.0504)
  point P102 (-16.3309, -14.1267)
  point P103 (-15.8182, -14.6961)
  point P104 (-14.6911, -14.2684)
  point P105 (-14.0232, -13.9088)
  point P106 (-13.6903, -13.674)
  point P107 (-13.0706, -14.2724)
  point P108 (-13.2937, -14.6133)
  point P109 (-13.6297, -15.2933)
  point P110 (-14.0178, -16.4347)
  point P111 (-13.4309, -16.9272)
  point P112 (-12.3742, -16.3468)
  point P113 (-11.7628, -15.8978)
  point P114 (-11.4659, -15.6189)
  point P115 (-10.7689, -16.1253)
  point P116 (-10.9425, -16.4939)
  point P117 (-11.1806, -17.2141)
  point P118 (-11.406, -18.3984)
  point P119 (-10.7563, -18.8044)
  point P120 (-9.7906, -18.0826)
  point P121 (-9.2477, -17.5529)
  point P122 (-8.9925, -17.2353)
  point P123 (-8.2318, -17.6398)
  point P124 (-8.3524, -18.0289)
  point P125 (-8.4879, -18.7753)
  point P126 (-8.5464, -19.9794)
  point P127 (-7.8464, -20.291)
  point P128 (-6.9907, -19.4419)
  point P129 (-6.5267, -18.8417)
  point P130 (-6.3182, -18.4918)
  point P131 (-5.5086, -18.7865)
  point P132 (-5.5738, -19.1886)
  point P133 (-5.6042, -19.9465)
  point P134 (-5.4945, -21.1471)
  point P135 (-4.758, -21.3583)
  point P136 (-3.6528, -19.7394)
  point P137 (-3.495, -19.3638)
  point P138 (-2.6523, -19.543)
  point P139 (-2.6609, -19.9502)
  point P140 (-2.5855, -20.705)
  point P141 (-2.3098, -21.8786)
  point P142 (-1.5511, -21.9853)
  point P143 (-0.9625, -20.9331)
  point P144 (-0.682, -20.2284)
  point P145 (0.2814, -19.8946)
  point P146 (0.3296, -20.2991)
  point P147 (0.5093, -21.036)
  point P148 (0.9457, -22.1599)
  point P149 (1.7119, -22.1599)
  point P150 (2.1483, -21.036)
  point P151 (2.328, -20.2991)
  point P152 (2.3762, -19.8946)
  point P153 (3.2356, -19.8345)
  point P154 (3.3396, -20.2284)
  point P155 (3.6201, -20.9331)
  point P156 (4.2087, -21.9853)
  point P157 (4.9674, -21.8786)
  point P158 (5.3185, -19.9502)
  point P159 (5.3099, -19.543)
  point P160 (6.1526, -19.3638)
  point P161 (6.3104, -19.7394)
  point P162 (6.6863, -20.3983)
  point P163 (7.4156, -21.3583)
  point P164 (8.1521, -21.1471)
  point P165 (8.2618, -19.9465)
  point P166 (8.2314, -19.1886)
  point P167 (8.1662, -18.7865)
  point P168 (8.9758, -18.4918)
  point P169 (9.1843, -18.8417)
  point P170 (9.6482, -19.4419)
  point P171 (10.504, -20.291)
  point P172 (11.2039, -19.9794)
  point P173 (11.1455, -18.7753)
  point P174 (11.0099, -18.0289)
  point P175 (10.8894, -17.6398)
  point P176 (11.6501, -17.2353)
  point P177 (11.9053, -17.5529)
  point P178 (12.4482, -18.0826)
  point P179 (13.4138, -18.8044)
  point P180 (14.0636, -18.3984)
  point P181 (13.8381, -17.2141)
  point P182 (13.6, -16.4939)
  point P183 (13.4265, -16.1253)
  point P184 (14.4204, -15.8978)
  point P185 (15.0318, -16.3468)
  point P186 (16.0885, -16.9272)
  point P187 (16.6754, -16.4347)
  point P188 (16.2873, -15.2933)
  point P189 (15.9513, -14.6133)
  point P190 (15.7282, -14.2724)
  point P191 (16.3479, -13.674)
  point P192 (16.6807, -13.9088)
  point P193 (17.3487, -14.2684)
  point P194 (18.4758, -14.6961)
  point P195 (18.9885, -14.1267)
  point P196 (18.4453, -13.0504)
  point P197 (18.0179, -12.4238)
  point P198 (17.7495, -12.1173)
  point P199 (18.6423, -11.6247)
  dimension "d2" = 360
  dimension "d4" = 5.98
  dimension "d5" = 3
  dimension "d7" = 4.5
  dimension "d8" = 2
  dimension "d11" = 360
  dimension "d13" = 0.05
  constraints: 801 point on circle, 401 centre point, 8 coincident, 2 tangent, 1 equal radius, 1511 other
  measures "d4" diameter of A360
  measures "d5" diameter of A361
  measures "d7" diameter of A362
  measures "d8" radius of A364
  measures "d13" radial gap between concentric circles of A378 A400
extrude "押し出し1" add sketch "スケッチ1" along normal blind 5 contours A1 A2 A359 A358 A355 A353 A352 A354 A356 A357 A351 A350 A347 A345 A344 A346 A348 A349 A343 A342 A339 A337 A336 A338 A340 A341 A335 A334 A331 A329 A328 A330 A332 A333 A327 A326 A323 A321 A320 A322 A324 A325 A319 A318 A315 A313 A312 A314 A316 A317 A311 A310 A307 A305 A304 A306 A308 A309 A303 A302 A299 A297 A296 A298 A300 A301 A295 A294 A291 A289 A288 A290 A292 A293 A287 A286 A283 A281 A280 A282 A284 A285 A279 A278 A275 A273 A272 A274 A276 A277 A271 A270 A267 A265 A264 A266 A268 A269 A263 A262 A259 A257 A256 A258 A260 A261 A255 A254 A251 A249 A248 A250 A252 A253 A247 A246 A243 A241 A240 A242 A244 A245 A239 A238 A235 A233 A232 A234 A236 A237 A231 A230 A227 A225 A224 A226 A228 A229 A223 A222 A219 A217 A216 A218 A220 A221 A215 A214 A211 A209 A208 A210 A212 A213 A207 A206 A203 A201 A200 A202 A204 A205 A199 A198 A195 A193 A192 A194 A196 A197 A191 A190 A187 A185 A184 A186 A188 A189 A183 A182 A179 A177 A176 A178 A180 A181 A175 A174 A171 A169 A168 A170 A172 A173 A167 A166 A163 A161 A160 A162 A164 A165 A159 A158 A155 A153 A152 A154 A156 A157 A151 A150 A147 A145 A144 A146 A148 A149 A143 A142 A139 A137 A136 A138 A140 A141 A135 A134 A131 A129 A128 A130 A132 A133 A127 A126 A123 A121 A120 A122 A124 A125 A119 A118 A115 A113 A112 A114 A116 A117 A111 A110 A107 A105 A104 A106 A108 A109 A103 A102 A99 A97 A96 A98 A100 A101 A95 A94 A91 A89 A88 A90 A92 A93 A87 A86 A83 A81 A80 A82 A84 A85 A79 A78 A75 A73 A72 A74 A76 A77 A71 A70 A67 A65 A64 A66 A68 A69 A63 A62 A59 A57 A56 A58 A60 A61 A55 A54 A51 A49 A48 A50 A52 A53 A47 A46 A43 A41 A40 A42 A44 A45 A39 A38 A35 A33 A32 A34 A36 A37 A31 A30 A27 A25 A24 A26 A28 A29 A23 A22 A19 A17 A16 A18 A20 A21 A15 A14 A11 A9 A8 A10 A12 A13 A7 A5 A4 A3 A6 A0
extrude "押し出し2" add sketch "スケッチ1" along normal blind 2.5 contours A365 A378 A374 A375 A377 A380 A370 A371 A373 A382 A366 A367 A369 A383 A364 A362 | A385 A400 A399 A398 A397 A396 A395 A394 A393 A392 A391 A390 A389 A388 A387 A386
sketch "スケッチ2" plane through (0, 0, 0) normal (0, 0, -1) x (-1, 0, 0)
  circle A0 centre (-6.7442, 7.4825) radius 1.5 projected
  circle A1 centre (-7.5526, -4.1567) radius 1.5 projected
  circle A2 centre (4.0866, -4.9652) radius 1.5 projected
  circle A3 centre (4.8951, 6.674) radius 1.5 projected
  circle A4 centre (-6.7442, 7.4825) radius 3.5
  circle A5 centre (4.8951, 6.674) radius 3.5
  circle A6 centre (-7.5526, -4.1567) radius 3.5
  circle A7 centre (4.0866, -4.9652) radius 3.5
  point P0 (0, 0)
  dimension "d18" = 7
  dimension "d19" = 7
  dimension "d21" = 7
  dimension "d22" = 7
  constraints: 4 centre point, 4 coincident
  measures "d18" diameter of A4
  measures "d19" diameter of A5
  measures "d21" diameter of A6
  measures "d22" diameter of A7
extrude "押し出し3" cut sketch "スケッチ2" against normal blind 0.8
